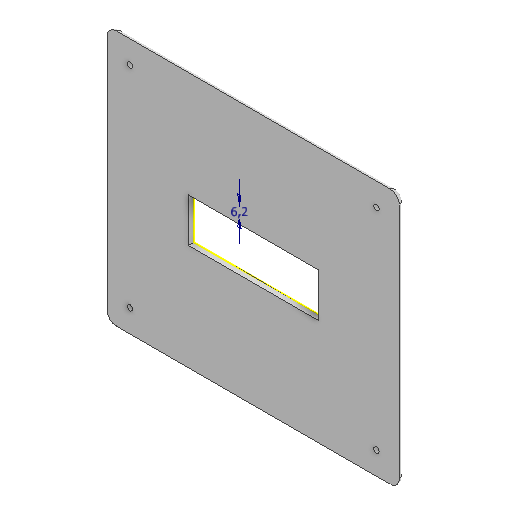
# Autodesk Inventor part: TutupBox
Saved by Autodesk Inventor 2026.2 (Build 302298010, 298A)
## iProperties
Created: 2026-05-29
Part Number: TutupBox
Material: Generic
Document SubType Name: Modeling
Designer: rizky
Density: 1 g/cm^3
Appearance: Default
Author: rizky
Autodesk Inventor part; units mm, degrees
ref_plane "YZ Plane" through (0, 0, 0) normal (1, 0, 0) x (0, 1, 0)
ref_plane "XZ Plane" through (0, 0, 0) normal (0, 1, 0) x (-1, 0, 0)
ref_plane "XY Plane" through (0, 0, 0) normal (0, 0, 1) x (1, 0, 0)
sketch "Sketch1" plane through (0, 0, 0) normal (0, 0, 1) x (1, 0, 0)
  line L0 (0, 0) -> (160, 0)
  line L1 (160, 0) -> (160, 140)
  line L2 (160, 140) -> (0, 140)
  line L3 (0, 140) -> (0, 0)
  dimension "d0" = 160
  dimension "d1" = 140
  constraints: 8 end point, 2 parallel, 1 horizontal, 1 perpendicular
  measures "d0" distance of L2.end L1.end
  measures "d1" distance of L1.end L0.end
extrude "Extrusion1" add sketch "Sketch1" along normal blind 3
fillet "Fillet1" radius 5 4 edges at (160, 140, 1.5) (0, 140, 1.5) (0, 0, 1.5) (160, 0, 1.5)
sketch "Sketch2" plane through (0, 0, 3) normal (0, 0, 1) x (1, 0, 0)
  arc A0 (155, 0) -> (160, 5) centre (155, 5) ccw projected
  line L0 (160, 5) -> (160, 135) projected
  arc A1 (160, 135) -> (155, 140) centre (155, 135) ccw projected
  line L1 (155, 140) -> (5, 140) projected
  arc A2 (5, 140) -> (0, 135) centre (5, 135) ccw projected
  line L2 (0, 135) -> (0, 5) projected
  arc A3 (0, 5) -> (5, 0) centre (5, 5) ccw projected
  line L3 (5, 0) -> (155, 0) projected
  line L4 (0, 0) -> (12.5, 0)
  line L5 (12.5, 0) -> (12.5, 12.5)
  line L6 (12.5, 12.5) -> (0, 12.5)
  line L7 (0, 12.5) -> (0, 0)
  circle A4 centre (12.5, 12.5) radius 1.5
  line L8 (80, 0) -> (80, 5)
  line L9 (0, 70) -> (5, 70)
  circle A5 centre (147.5, 12.5) radius 1.5
  circle A6 centre (12.5, 127.5) radius 1.5
  circle A7 centre (147.5, 127.5) radius 1.5
  dimension "d5" = 12.5
  dimension "d6" = 12.5
  dimension "d7" = 3
  dimension "d8" = 5
  dimension "d9" = 5
  constraints: 12 end point, 4 centre point, 3 symmetric about line, 2 horizontal, 2 midpoint, 2 parallel, 1 coincident, 1 perpendicular, 1 vertical, 3 other
  measures "d5" distance of L6.end L5.end
  measures "d6" distance of L5.end L4.end
  measures "d7" diameter of A4
  measures "d8" distance of L8.start L8.end
  measures "d9" distance of L9.start L9.end
extrude "Extrusion2" cut sketch "Sketch2" against normal through all contours A4 L6 L5 | L5 L6 A4 | A5 | A6 | A7
fillet "Fillet2" radius 3 8 edges at (1.4645, 138.5355, 0) (0, 70, 0) (1.4645, 1.4645, 0) (80, 0, 0) (158.5355, 1.4645, 0) (160, 70, 0) (158.5355, 138.5355, 0) (80, 140, 0)
sketch "Sketch3" plane through (0, 0, 0) normal (0, 0, -1) x (-1, 0, 0)
  line L0 (-155, 140) -> (-5, 140) projected
  line L1 (-5, 0) -> (-155, 0) projected
  line L2 (-160, 5) -> (-160, 135) projected
  line L3 (0, 135) -> (0, 5) projected
  line L4 (-80, 0) -> (-80, 58)
  line L5 (-80, 58) -> (-115.5, 58)
  line L6 (-115.5, 58) -> (-115.5, 82)
  line L7 (-115.5, 82) -> (-80, 82)
  line L8 (-80, 82) -> (-80, 58)
  line L9 (-80, 58) -> (-44.5, 58)
  line L10 (-44.5, 58) -> (-44.5, 82)
  line L11 (-44.5, 82) -> (-80, 82)
  point P0 (0, 0)
  dimension "d13" = 58
  dimension "d14" = 35.5
  dimension "d15" = 24
  constraints: 16 end point, 2 parallel, 2 symmetric about line, 1 horizontal, 1 midpoint, 1 perpendicular, 1 vertical
  measures "d13" distance of L4.start L4.end
  measures "d14" distance of L6.end L7.end
  measures "d15" distance of L5.end L6.end
extrude "Extrusion3" cut sketch "Sketch3" against normal blind 10
sketch "Sketch4" plane through (0, 0, 0) normal (0, 0, -1) x (-1, 0, 0)
  line L0 (-44.5, 58) -> (-115.5, 58) projected
  line L1 (-115.5, 58) -> (-115.5, 82) projected
  line L2 (-115.5, 82) -> (-44.5, 82) projected
  line L3 (-44.5, 82) -> (-44.5, 58) projected
  circle A0 centre (-12.5, 127.5) radius 1.5 projected
  circle A1 centre (-147.5, 12.5) radius 1.5 projected
  circle A2 centre (-147.5, 127.5) radius 1.5 projected
  circle A3 centre (-12.5, 12.5) radius 1.5 projected
  arc A4 (-3, 135) -> (-5, 137) centre (-5, 135) ccw projected
  line L4 (-155, 137) -> (-5, 137) projected
  arc A5 (-155, 137) -> (-157, 135) centre (-155, 135) ccw projected
  line L5 (-157, 5) -> (-157, 135) projected
  arc A6 (-157, 5) -> (-155, 3) centre (-155, 5) ccw projected
  line L6 (-5, 3) -> (-155, 3) projected
  arc A7 (-5, 3) -> (-3, 5) centre (-5, 5) ccw projected
  line L7 (-3, 135) -> (-3, 5) projected
  line L8 (-119.0625, 88.2) -> (-28.575, 88.2)
  point P0 (0, 0)
  dimension "d18" = 6.2
  constraints: 2 end point, 1 horizontal
  measures "d18" distance between parallel lines of L2 L8
body "Solid1"
